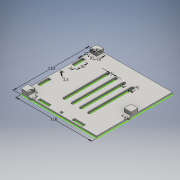
# Autodesk Inventor part: base_agitador
Saved by Autodesk Inventor 2016 (Build 200138000, 138)
## iProperties
Created: 2016-05-22
Part Number: base_agitador
Material: Generic
Document SubType Name: Modeling
Designer: JV
Density: 1 g/cm^3
Appearance: Default
Author: JV
Autodesk Inventor part; units mm, degrees
ref_plane "YZ Plane" through (0, 0, 0) normal (1, 0, 0) x (0, 1, 0)
ref_plane "XZ Plane" through (0, 0, 0) normal (0, 1, 0) x (-1, 0, 0)
ref_plane "XY Plane" through (0, 0, 0) normal (0, 0, 1) x (1, 0, 0)
sketch "Sketch1" plane through (0, 0, 0) normal (0, 0, 1) x (1, 0, 0)
  line L0 (-0.1956, -75.4616) -> (-110.1956, -75.4616)
  line L1 (-110.1956, -75.4616) -> (-110.1956, 34.5384)
  line L2 (-110.1956, 34.5384) -> (-0.1956, 34.5384)
  line L3 (-110.1956, 34.5384) -> (-108.1956, 34.5384) construction
  line L4 (-108.1956, 12.5384) -> (-104.1956, 12.5384)
  line L5 (-104.1956, 12.5384) -> (-104.1956, -3.4616)
  line L6 (-104.1956, -3.4616) -> (-108.1956, -3.4616)
  line L7 (-108.1956, -3.4616) -> (-108.1956, 12.5384)
  line L8 (-110.1956, 34.5384) -> (-110.1956, 32.5384) construction
  line L9 (-110.1956, -20.4616) -> (-0.1956, -20.4616) construction
  line L10 (-108.1956, -53.4616) -> (-104.1956, -53.4616)
  line L11 (-104.1956, -53.4616) -> (-104.1956, -37.4616)
  line L12 (-104.1956, -37.4616) -> (-108.1956, -37.4616)
  line L13 (-108.1956, -37.4616) -> (-108.1956, -53.4616)
  line L14 (-88.1956, -73.4616) -> (-72.1956, -73.4616)
  line L15 (-72.1956, -73.4616) -> (-72.1956, -69.4616)
  line L16 (-72.1956, -69.4616) -> (-88.1956, -69.4616)
  line L17 (-88.1956, -69.4616) -> (-88.1956, -73.4616)
  line L18 (-22.1956, -73.4616) -> (-38.1956, -73.4616)
  line L19 (-38.1956, -73.4616) -> (-38.1956, -69.4616)
  line L20 (-38.1956, -69.4616) -> (-22.1956, -69.4616)
  line L21 (-22.1956, -69.4616) -> (-22.1956, -73.4616)
  circle A0 centre (-55.1956, -71.4616) radius 1.75
  circle A1 centre (-106.1956, -20.4616) radius 1.75
  line L22 (-0.1956, 34.5384) -> (-0.1956, -75.4616)
  line L23 (-110.1956, 34.5384) -> (-100.1956, 34.5384)
  line L24 (-100.1956, 34.5384) -> (-100.1956, 24.5384)
  line L25 (-100.1956, 24.5384) -> (-110.1956, 24.5384)
  line L26 (-110.1956, 24.5384) -> (-110.1956, 34.5384)
  line L27 (-0.1956, -25.4616) -> (-10.1956, -25.4616)
  line L28 (-10.1956, -25.4616) -> (-10.1956, -15.4616)
  line L29 (-10.1956, -15.4616) -> (-0.1956, -15.4616)
  line L30 (-72.5638, 12.5384) -> (-68.5638, 12.5384)
  line L31 (-68.5638, 12.5384) -> (-68.5638, -53.4616)
  line L32 (-68.5638, -53.4616) -> (-72.5638, -53.4616)
  line L33 (-72.5638, -53.4616) -> (-72.5638, 12.5384)
  line L34 (-60.5638, 12.5384) -> (-60.5638, -53.4616)
  line L35 (-56.5638, 12.5384) -> (-56.5638, -53.4616)
  line L36 (-48.5638, 12.5384) -> (-48.5638, -53.4616)
  line L37 (-44.5638, 12.5384) -> (-44.5638, -53.4616)
  line L38 (-36.5638, 12.5384) -> (-36.5638, -53.4616)
  line L39 (-32.5638, 12.5384) -> (-32.5638, -53.4616)
  line L40 (-60.5638, -53.4616) -> (-56.5638, -53.4616)
  line L41 (-48.5638, -53.4616) -> (-44.5638, -53.4616)
  line L42 (-36.5638, -53.4616) -> (-32.5638, -53.4616)
  line L43 (-60.5638, 12.5384) -> (-56.5638, 12.5384)
  line L44 (-48.5638, 12.5384) -> (-44.5638, 12.5384)
  line L45 (-36.5638, 12.5384) -> (-32.5638, 12.5384)
  line L46 (-110.1956, -75.4616) -> (-100.1956, -75.4616)
  line L47 (-100.1956, -75.4616) -> (-100.1956, -65.4616)
  line L48 (-100.1956, -65.4616) -> (-110.1956, -65.4616)
  line L49 (-110.1956, -65.4616) -> (-110.1956, -75.4616)
  dimension "d5" = 110
  dimension "d6" = 110
  dimension "d7" = 2
  dimension "d8" = 22
  dimension "d10" = 4
  dimension "d11" = 16
  dimension "d12" = 2
  dimension "d20" = 3.5
  dimension "d21" = 10
  dimension "d22" = 10
  dimension "d25" = 10
  dimension "d26" = 4
  dimension "d30" = 4
  dimension "d33" = 4
  dimension "d34" = 4
  dimension "d35" = 4
  dimension "d37" = 10
  dimension "d38" = 10
  constraints: 100 end point, 12 equal length, 10 horizontal, 5 perpendicular, 5 point on line, 4 symmetric about line, 3 vertical, 2 centre point, 1 midpoint
  measures "d5" distance of L0.start L0.end
  measures "d6" distance of L0.end L1.end
  measures "d7" distance of L1.end L3.end
  measures "d8" distance of L3.end L4.start
  measures "d10" distance of L5.end L6.end
  measures "d11" distance of L4.end L5.end
  measures "d12" distance of L1.end L8.end
  measures "d20" diameter of A1
  measures "d21" distance of L24.end L25.end
  measures "d22" distance of L23.end L24.end
  measures "d25" distance of L27.start L27.end
  measures "d26" distance of L30.start L30.end
  measures "d30" distance of L36.start L37.start
  measures "d33" distance of L38.start L39.start
  measures "d34" distance of L39.start L38.start
  measures "d35" distance of L38.start L39.start
  measures "d37" distance of L48.end L47.end
  measures "d38" distance of L47.end L46.end
extrude "Extrusion3" add sketch "Sketch1" along normal blind 3 contours L0 L47 L48 L1 L25 L24 L2 L22 L29 L28 L27
extrude "Extrusion4" add sketch "Sketch1" along normal blind 8 contours L0 L1 L48 L47 | L27 L28 L29 L22 | L1 L2 L24 L25
fillet "Fillet1" radius 3 1 edges at (-110.1956, 34.5384, 4)
fillet "Fillet2" radius 2 1 edges at (-110.1956, -75.4616, 4)
fillet "Fillet3" radius 2 16 edges at (-32.5638, 12.5384, 1.5) (-36.5638, 12.5384, 1.5) (-48.5638, 12.5384, 1.5) (-44.5638, 12.5384, 1.5) (-56.5638, 12.5384, 1.5) (-68.5638, 12.5384, 1.5) (-60.5638, 12.5384, 1.5) (-72.5638, 12.5384, 1.5) (-68.5638, -53.4616, 1.5) (-72.5638, -53.4616, 1.5) (-60.5638, -53.4616, 1.5) (-56.5638, -53.4616, 1.5) (-48.5638, -53.4616, 1.5) (-44.5638, -53.4616, 1.5) (-36.5638, -53.4616, 1.5) (-32.5638, -53.4616, 1.5)
body "Solid2"
